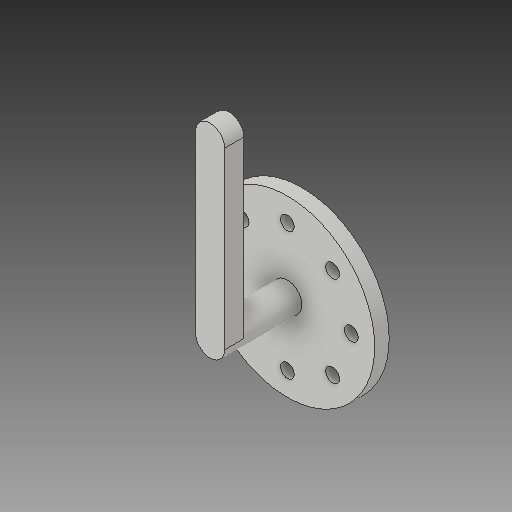
# Autodesk Inventor part: pin holder
Saved by Autodesk Inventor 2018.1 (Build 221171000, 171)
## iProperties
Created: 2017-08-02
Part Number: pin holder
Material: Generic
Document SubType Name: Modeling
Designer: Kai
Density: 1 g/cm^3
Appearance: Default
Author: Kai
Autodesk Inventor part; units mm, degrees
ref_plane "YZ Plane" through (0, 0, 0) normal (1, 0, 0) x (0, 1, 0)
ref_plane "XZ Plane" through (0, 0, 0) normal (0, 1, 0) x (-1, 0, 0)
ref_plane "XY Plane" through (0, 0, 0) normal (0, 0, 1) x (1, 0, 0)
sketch "Sketch1" plane through (0, 0, 0) normal (0, 0, 1) x (1, 0, 0)
  circle A0 centre (0, 0) radius 38.1
  circle A1 centre (0, 0) radius 27.94 construction
  circle A2 centre (0, 27.94) radius 3
  circle A3 centre (0, 0) radius 27.94 construction
  circle A4 centre (-19.7566, 19.7566) radius 3
  circle A5 centre (0, 0) radius 27.94 construction
  circle A6 centre (-27.94, 0) radius 3
  circle A7 centre (0, 0) radius 27.94 construction
  circle A8 centre (-19.7566, -19.7566) radius 3
  circle A9 centre (0, 0) radius 27.94 construction
  circle A10 centre (0, -27.94) radius 3
  circle A11 centre (0, 0) radius 27.94 construction
  circle A12 centre (19.7566, -19.7566) radius 3
  circle A13 centre (0, 0) radius 27.94 construction
  circle A14 centre (27.94, 0) radius 3
  circle A15 centre (0, 0) radius 27.94 construction
  circle A16 centre (19.7566, 19.7566) radius 3
  dimension "d1" = 55.88
  dimension "d0" = 76.2
  dimension "d2" = 6
  dimension "d5" = 360
  constraints: 9 centre point, 2 coincident, 2 horizontal alignment, 2 vertical alignment, 53 other
  measures "d0" diameter of A0
  measures "d2" diameter of A2
extrude "Extrusion1" add sketch "Sketch1" along normal blind 6.35
sketch "Sketch2" plane through (0, 0, 6.35) normal (0, 0, 1) x (1, 0, 0)
  circle A0 centre (0, 0) radius 6.35
  dimension "d9" = 12.7
  constraints: 1 centre point, 1 coincident
  measures "d9" diameter of A0
extrude "Extrusion2" add sketch "Sketch2" along normal blind 25.4
sketch "Sketch3" plane through (0, 0, 31.75) normal (0, 0, 1) x (1, 0, 0)
  arc A0 (-6.35, 0) -> (6.35, 0) centre (0, 0) ccw
  line L0 (6.35, 0) -> (6.35, 76.2397)
  line L1 (-6.35, 0) -> (-6.35, 76.2397)
  arc A1 (6.35, 76.2397) -> (-6.35, 76.2397) centre (0, 76.2397) ccw
  constraints: 4 end point, 4 point on circle, 2 centre point, 2 vertical, 1 coincident, 1 tangent
extrude "Extrusion3" add sketch "Sketch3" along normal blind 8.382
body "Solid1"
